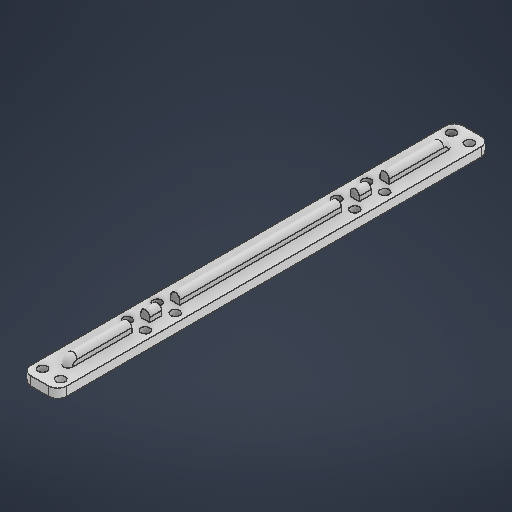
# Autodesk Inventor part: structural_bar1
Saved by Autodesk Inventor 2026.1 (Build 301233000, 233)
## iProperties
Created: 2026-05-17
Part Number: structural_bar1
Material: Generic
Document SubType Name: Modeling
Designer: emanuel
Density: 1 g/cm^3
Appearance: Default
Author: emanuel
Autodesk Inventor part; units mm, degrees
ref_plane "YZ Plane" through (0, 0, 0) normal (1, 0, 0) x (0, 1, 0)
ref_plane "XZ Plane" through (0, 0, 0) normal (0, 1, 0) x (-1, 0, 0)
ref_plane "XY Plane" through (0, 0, 0) normal (0, 0, 1) x (1, 0, 0)
sketch "Sketch1" plane through (0, 0, 0) normal (0, 1, 0) x (-1, 0, 0)
  line L0 (0, 0) -> (12, 0)
  line L1 (12, 0) -> (12, -144.6)
  line L2 (12, -144.6) -> (0, -144.6)
  line L3 (0, -144.6) -> (0, 0)
  line L4 (0, 0) -> (3, 0)
  line L5 (3, 0) -> (3, -4)
  line L6 (3, -4) -> (0, -4)
  line L7 (0, -4) -> (0, 0)
  line L8 (3, -4) -> (9, -4)
  circle A0 centre (9, -4) radius 1.5
  circle A1 centre (3, -4) radius 1.5
  line L9 (12, -144.6) -> (9, -144.6)
  line L10 (9, -144.6) -> (9, -140.6)
  line L11 (9, -140.6) -> (12, -140.6)
  line L12 (12, -140.6) -> (12, -144.6)
  line L13 (9, -140.6) -> (3, -140.6)
  circle A2 centre (9, -140.6) radius 1.5
  circle A3 centre (3, -140.6) radius 1.5
  dimension "d0" = 12
  dimension "d1" = 144.6
  dimension "d2" = 3
  dimension "d3" = 4
  dimension "d4" = 6
  dimension "d5" = 3
  dimension "d6" = 3
  dimension "d7" = 3
  dimension "d8" = 4
  dimension "d9" = 6
  dimension "d10" = 3
  dimension "d11" = 3
  constraints: 28 end point, 6 parallel, 5 horizontal, 4 centre point, 4 coincident, 3 perpendicular
  measures "d0" distance of L1.end L2.end
  measures "d1" distance of L0.end L1.end
  measures "d2" distance of L5.end L6.end
  measures "d3" distance of L4.end L5.end
  measures "d4" distance of L5.end L8.end
  measures "d5" diameter of A0
  measures "d6" diameter of A1
  measures "d7" distance of L10.end L11.end
  measures "d8" distance of L9.end L10.end
  measures "d9" distance of L10.end L13.end
  measures "d10" diameter of A2
  measures "d11" diameter of A3
extrude "Extrusion1" add sketch "Sketch1" along normal blind 3 contours L0 L5 A1 L6 L3 | L0 L1 L11 A2 L10 L2 L3 L6 A1 L5 | L1 L2 L10 A2 L11
sketch "Sketch2" plane through (0, 3, 0) normal (0, 1, 0) x (1, 0, 0)
  line L0 (-12, 0) -> (0, 0) projected
  line L1 (-6, 0) -> (-6, 144.6) construction
  line L2 (0, 144.6) -> (-12, 144.6) projected
  line L3 (-4.5, 0) -> (-4.5, 144.6)
  line L4 (-7.5, 144.6) -> (-7.5, 0)
  arc A0 (-7.5, 0) -> (-4.5, 0) centre (-6, 0) ccw
  arc A1 (-4.5, 144.6) -> (-7.5, 144.6) centre (-6, 144.6) ccw
  line L5 (0, 0) -> (0, 144.6) projected
  line L6 (-12, 0) -> (0, 0)
  line L7 (0, 0) -> (0, 8)
  line L8 (0, 8) -> (-12, 8)
  line L9 (-12, 8) -> (-12, 0)
  line L10 (-12, 144.6) -> (0, 144.6)
  line L11 (0, 144.6) -> (0, 136.6)
  line L12 (0, 136.6) -> (-12, 136.6)
  line L13 (-12, 136.6) -> (-12, 144.6)
  point P0 (-6, 72.3)
  point P1 (-4.5, 136.6)
  point P2 (-7.5, 136.6)
  point P3 (-7.5, 8)
  point P4 (-4.5, 8)
  dimension "d14" = 3
  dimension "d15" = 8
  dimension "d16" = 8
  constraints: 24 end point, 5 parallel, 4 point on circle, 4 tangent, 3 midpoint, 2 centre point, 2 horizontal, 2 perpendicular, 2 point on line
  measures "d14" diameter of A1
  measures "d15" distance of L7.end L6.end
  measures "d16" distance of L10.end L11.end
extrude "Extrusion2" add sketch "Sketch2" along normal blind 3 contours L4 L12 L3 L8
fillet "Fillet1" radius 3 2 edges at (-6, 6, -8) (-6, 6, -136.6)
fillet "Fillet2" radius 3 4 edges at (0, 1.5, 0) (-12, 1.5, 0) (-12, 1.5, -144.6) (0, 1.5, -144.6)
fillet "Fillet3" radius 1.5 6 edges at (-7.5, 5.1215, -8.8785) (-7.5, 5.1215, -135.7215) (-7.5, 6, -72.3) (-4.5, 5.1215, -135.7215) (-4.5, 5.1215, -8.8785) (-4.5, 6, -72.3)
sketch "Sketch3" plane through (0, 3, 0) normal (0, 1, 0) x (1, 0, 0)
  line L0 (-12, 141.6) -> (-12, 3) projected
  line L1 (-12, 72.3) -> (-6, 72.3)
  line L2 (-9, 42.3) -> (-3, 42.3)
  line L3 (-3, 42.3) -> (-3, 102.3)
  line L4 (-3, 102.3) -> (-9, 102.3)
  line L5 (-9, 102.3) -> (-9, 42.3)
  line L6 (-9, 42.3) -> (-3, 102.3) construction
  line L7 (-3, 42.3) -> (-9, 102.3) construction
  line L8 (-9, 32.3) -> (-3, 32.3)
  line L9 (-3, 32.3) -> (-3, 112.3)
  line L10 (-3, 112.3) -> (-9, 112.3)
  line L11 (-9, 112.3) -> (-9, 32.3)
  line L12 (-9, 32.3) -> (-3, 112.3) construction
  line L13 (-3, 32.3) -> (-9, 112.3) construction
  line L14 (-9, 112.3) -> (-3, 112.3) construction
  line L15 (-9, 109.3) -> (-3, 109.3)
  line L16 (-3, 115.3) -> (-9, 115.3)
  arc A0 (-9, 115.3) -> (-9, 109.3) centre (-9, 112.3) ccw
  arc A1 (-3, 109.3) -> (-3, 115.3) centre (-3, 112.3) ccw
  circle A2 centre (-9, 112.3) radius 1.5
  circle A3 centre (-3, 112.3) radius 1.5
  circle A4 centre (-9, 102.3) radius 1.5
  circle A5 centre (-3, 102.3) radius 1.5
  line L17 (-9, 102.3) -> (-3, 102.3) construction
  line L18 (-9, 99.3) -> (-3, 99.3)
  line L19 (-3, 105.3) -> (-9, 105.3)
  arc A6 (-9, 105.3) -> (-9, 99.3) centre (-9, 102.3) ccw
  arc A7 (-3, 99.3) -> (-3, 105.3) centre (-3, 102.3) ccw
  line L20 (-3, 32.3) -> (-9, 32.3)
  line L21 (-3, 42.3) -> (-9, 42.3)
  line L22 (-9, 42.3) -> (-3, 42.3) construction
  line L23 (-9, 39.3) -> (-3, 39.3)
  line L24 (-3, 45.3) -> (-9, 45.3)
  arc A8 (-9, 45.3) -> (-9, 39.3) centre (-9, 42.3) ccw
  arc A9 (-3, 39.3) -> (-3, 45.3) centre (-3, 42.3) ccw
  circle A10 centre (-9, 42.3) radius 1.5
  circle A11 centre (-3, 42.3) radius 1.5
  circle A12 centre (-9, 32.3) radius 1.5
  circle A13 centre (-3, 32.3) radius 1.5
  line L25 (-9, 32.3) -> (-3, 32.3) construction
  line L26 (-9, 29.3) -> (-3, 29.3)
  line L27 (-3, 35.3) -> (-9, 35.3)
  arc A14 (-9, 35.3) -> (-9, 29.3) centre (-9, 32.3) ccw
  arc A15 (-3, 29.3) -> (-3, 35.3) centre (-3, 32.3) ccw
  point P0 (0, 0)
  point P1 (-6, 112.3)
  point P2 (-6, 102.3)
  point P3 (-6, 42.3)
  point P4 (-6, 32.3)
  dimension "d22" = 6
  dimension "d23" = 6
  dimension "d24" = 60
  dimension "d25" = 6
  dimension "d26" = 80
  dimension "d27" = 6
  dimension "d28" = 3
  dimension "d29" = 3
  dimension "d30" = 3
  dimension "d31" = 3
  dimension "d32" = 6
  dimension "d33" = 6
  dimension "d34" = 6
  dimension "d35" = 6
  dimension "d36" = 3
  dimension "d37" = 3
  dimension "d38" = 3
  dimension "d39" = 3
  dimension "d40" = 6
  constraints: 62 end point, 16 centre point, 16 point on circle, 16 tangent, 12 equal length, 9 midpoint, 8 coincident, 3 horizontal, 2 perpendicular
  measures "d22" distance of L1.start L1.end
  measures "d23" distance of L4.end L3.end
  measures "d24" distance of L3.end L2.end
  measures "d25" distance of L10.end L9.end
  measures "d26" distance of L9.end L8.end
  measures "d27" diameter of A1
  measures "d28" diameter of A2
  measures "d29" diameter of A3
  measures "d30" diameter of A4
  measures "d31" diameter of A5
  measures "d32" diameter of A7
  measures "d33" distance of L20.end L20.start
  measures "d34" distance of L21.end L21.start
  measures "d35" diameter of A9
  measures "d36" diameter of A10
  measures "d37" diameter of A11
  measures "d38" diameter of A12
  measures "d39" diameter of A13
  measures "d40" diameter of A15
extrude "Extrusion3" cut sketch "Sketch3" along normal blind 3 contours A0 L16 A1 L9 A3 L10 A2 L11 | A6 L11 A4 L5 | L11 A2 L10 A3 L9 L15 | L19 L9 A5 L4 A4 L11 | L5 A4 L4 A5 L3 L18 | A8 L5 A10 L11 | A7 L3 A5 L9 | A14 L11 A12 L8 A13 L9 A15 L26 | L24 L3 A11 L2 A10 L5 | L11 A10 L2 A11 L9 L23 | A9 L9 A11 L3 | L27 L9 A13 L8 A12 L11
extrude "Extrusion4" cut sketch "Sketch3" against normal blind 3 contours A2 L10 L11 | L11 L10 A2 | A4 L4 L11 | L11 L5 A4 | L5 L4 A4 | A3 L10 L9 | L9 L10 A3 | A5 L3 L9 | L9 L4 A5 | A5 L4 L3 | A10 L2 L5 | L5 L11 A10 | L11 L2 A10 | A11 L9 L3 | L3 L2 A11 | A12 L8 L11 | L11 L8 A12 | A11 L2 L9 | A13 L8 L9 | L9 L8 A13
body "Solid1"
